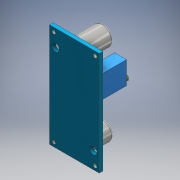
# Autodesk Inventor part: pcb_with_elements
Saved by Autodesk Inventor 2016 (Build 200138000, 138)
## iProperties
Created: 2016-10-13
Part Number: pcb_with_elements
Material: Generic
Document SubType Name: Modeling
Designer: Jakub
Density: 1 g/cm^3
Appearance: Default
Mass: 4.43836 g
Surface Area: 33.9944 cm^2
Volume: 4.43836 cm^3
Author: Jakub
Autodesk Inventor part; units mm, degrees
ref_plane "YZ Plane" through (0, 0, 0) normal (1, 0, 0) x (0, 1, 0)
ref_plane "XZ Plane" through (0, 0, 0) normal (0, 1, 0) x (-1, 0, 0)
ref_plane "XY Plane" through (0, 0, 0) normal (0, 0, 1) x (1, 0, 0)
sketch "Sketch1" plane through (0, 0, 0) normal (0, 1, 0) x (-1, 0, 0)
  line L0 (-10.375, 21.675) -> (10.375, 21.675)
  line L1 (10.375, 21.675) -> (10.375, -21.675)
  line L2 (10.375, -21.675) -> (-10.375, -21.675)
  line L3 (-10.375, -21.675) -> (-10.375, 21.675)
  line L4 (-10.375, 21.675) -> (10.375, -21.675) construction
  line L5 (10.375, 21.675) -> (-10.375, -21.675) construction
  point P0 (0, 0)
  dimension "d0" = 20.75
  dimension "d1" = 43.35
  constraints: 12 end point, 2 midpoint, 2 parallel, 1 horizontal, 1 perpendicular
  measures "d0" distance of L1.end L2.end
  measures "d1" distance of L0.end L1.end
extrude "Extrusion1" add sketch "Sketch1" along normal blind 1.5
sketch "Sketch2" plane through (0, 1.5, 0) normal (0, 1, 0) x (1, 0, 0)
  circle A0 centre (-8.625, -19.925) radius 0.75
  circle A1 centre (-8.625, 19.925) radius 0.75
  circle A2 centre (8.625, -19.925) radius 0.75
  circle A3 centre (8.625, 19.925) radius 0.75
  line L0 (-10.375, -21.675) -> (10.375, -21.675) projected
  line L1 (10.375, -21.675) -> (10.375, 21.675) projected
  line L2 (-10.375, 21.675) -> (-10.375, -21.675) projected
  line L3 (10.375, 21.675) -> (-10.375, 21.675) projected
  point P0 (0, 0)
  dimension "d4" = 1.5
  dimension "d5" = 1.5
  dimension "d6" = 1.5
  dimension "d7" = 1.5
  dimension "d8" = 1.75
  dimension "d9" = 1.75
  dimension "d10" = 1.75
  dimension "d11" = 1.75
  dimension "d12" = 1.75
  dimension "d13" = 1.75
  dimension "d14" = 1.75
  dimension "d15" = 1.75
  constraints: 4 centre point
  measures "d4" diameter of A0
  measures "d5" diameter of A1
  measures "d6" diameter of A2
  measures "d7" diameter of A3
  measures "d8" distance from line of L0 A2.centre
  measures "d9" distance from line of L1 A2.centre
  measures "d10" distance from line of L0 A0.centre
  measures "d11" distance from line of L2 A0.centre
  measures "d12" distance from line of L3 A1.centre
  measures "d13" distance from line of L2 A1.centre
  measures "d14" distance from line of L1 A3.centre
  measures "d15" distance from line of L3 A3.centre
extrude "Extrusion2" cut sketch "Sketch2" against normal up to next contours A0 | A1 | A2 | A3
sketch "Sketch3" plane through (0, 1.5, 0) normal (0, 1, 0) x (1, 0, 0)
  circle A0 centre (7.875, 14.675) radius 1.5
  circle A1 centre (-7.875, -14.675) radius 1.5
  line L0 (-10.375, 21.675) -> (-10.375, -21.675) projected
  line L1 (10.375, 21.675) -> (10.375, -21.675) projected
  line L2 (10.375, 21.675) -> (-10.375, 21.675) projected
  line L3 (-10.375, -21.675) -> (10.375, -21.675) projected
  point P0 (0, 0)
  dimension "d18" = 3
  dimension "d19" = 3
  dimension "d20" = 2.5
  dimension "d21" = 2.5
  dimension "d22" = 7
  dimension "d23" = 7
  constraints: 2 centre point
  measures "d18" diameter of A0
  measures "d19" diameter of A1
  measures "d20" distance from line of L0 A1.centre
  measures "d21" distance from line of L1 A0.centre
  measures "d22" distance from line of L2 A0.centre
  measures "d23" distance from line of L3 A1.centre
extrude "Extrusion3" cut sketch "Sketch3" against normal up to next contours A0 | A1
sketch "Sketch4" plane through (0, 1.5, 0) normal (0, 1, 0) x (1, 0, 0)
  line L0 (-7.125, -18.425) -> (-10.125, -18.425)
  line L1 (-10.125, -18.425) -> (-10.125, -21.425)
  line L2 (-10.125, -21.425) -> (-7.125, -21.425)
  line L3 (-7.125, -21.425) -> (-7.125, -18.425)
  circle A0 centre (-8.625, -19.925) radius 0.75 projected
  line L4 (-7.125, -18.425) -> (-10.125, -21.425) construction
  line L5 (-10.125, -18.425) -> (-7.125, -21.425) construction
  line L6 (10.125, -21.425) -> (7.125, -21.425)
  line L7 (7.125, -21.425) -> (7.125, -18.425)
  line L8 (7.125, -18.425) -> (10.125, -18.425)
  line L9 (10.125, -18.425) -> (10.125, -21.425)
  circle A1 centre (8.625, -19.925) radius 0.75 projected
  line L10 (10.125, -21.425) -> (7.125, -18.425) construction
  line L11 (7.125, -21.425) -> (10.125, -18.425) construction
  line L12 (7.125, 18.425) -> (10.125, 18.425)
  line L13 (10.125, 18.425) -> (10.125, 21.425)
  line L14 (10.125, 21.425) -> (7.125, 21.425)
  line L15 (7.125, 21.425) -> (7.125, 18.425)
  circle A2 centre (8.625, 19.925) radius 0.75 projected
  line L16 (7.125, 18.425) -> (10.125, 21.425) construction
  line L17 (10.125, 18.425) -> (7.125, 21.425) construction
  line L18 (-10.125, 21.425) -> (-7.125, 21.425)
  line L19 (-7.125, 21.425) -> (-7.125, 18.425)
  line L20 (-7.125, 18.425) -> (-10.125, 18.425)
  line L21 (-10.125, 18.425) -> (-10.125, 21.425)
  circle A3 centre (-8.625, 19.925) radius 0.75 projected
  line L22 (-10.125, 21.425) -> (-7.125, 18.425) construction
  line L23 (-7.125, 21.425) -> (-10.125, 18.425) construction
  circle A4 centre (-8.625, -19.925) radius 0.75
  circle A5 centre (8.625, -19.925) radius 0.75
  circle A6 centre (-8.625, 19.925) radius 0.75
  circle A7 centre (8.625, 19.925) radius 0.75
  point P0 (0, 0)
  dimension "d26" = 3
  dimension "d27" = 3
  dimension "d28" = 3
  dimension "d29" = 3
  dimension "d30" = 3
  dimension "d31" = 3
  dimension "d32" = 3
  dimension "d33" = 3
  constraints: 48 end point, 8 midpoint, 8 parallel, 4 centre point, 4 coincident, 4 concentric, 4 horizontal, 4 perpendicular
  measures "d26" distance of L2.end L1.end
  measures "d27" distance of L1.end L0.end
  measures "d28" distance of L7.end L8.end
  measures "d29" distance of L6.end L7.end
  measures "d30" distance of L14.end L13.end
  measures "d31" distance of L13.end L12.end
  measures "d32" distance of L19.end L20.end
  measures "d33" distance of L18.end L19.end
extrude "Extrusion4" add sketch "Sketch4" along normal blind 0.01
sketch "Sketch5" plane through (0, 1.5, 0) normal (0, 1, 0) x (1, 0, 0)
  circle A0 centre (0, 17.175) radius 4
  line L0 (10.375, 21.675) -> (-10.375, 21.675) projected
  point P0 (0, 0)
  dimension "d36" = 8
  dimension "d37" = 4.5
  constraints: 1 centre point
  measures "d36" diameter of A0
  measures "d37" distance from line of L0 A0.centre
extrude "Extrusion5" add sketch "Sketch5" along normal blind 11
sketch "Sketch6" plane through (0, 1.5, 0) normal (0, 1, 0) x (1, 0, 0)
  circle A0 centre (0, -17.175) radius 4
  line L0 (-10.375, -21.675) -> (10.375, -21.675) projected
  point P0 (0, 0)
  dimension "d40" = 8
  dimension "d41" = 4.5
  constraints: 1 centre point
  measures "d40" diameter of A0
  measures "d41" distance from line of L0 A0.centre
extrude "Extrusion6" add sketch "Sketch6" along normal blind 11
sketch "Sketch7" plane through (0, 1.5, 0) normal (0, 1, 0) x (1, 0, 0)
  line L0 (2.125, -12.175) -> (-9.875, -12.175)
  line L1 (-9.875, -12.175) -> (-9.875, -0.175)
  line L2 (-9.875, -0.175) -> (2.125, -0.175)
  line L3 (2.125, -0.175) -> (2.125, -12.175)
  line L4 (2.125, -12.175) -> (-9.875, -0.175) construction
  line L5 (-9.875, -12.175) -> (2.125, -0.175) construction
  line L6 (-10.375, 21.675) -> (-10.375, -21.675) projected
  circle A0 centre (0, -17.175) radius 4 projected
  point P0 (0, 0)
  point P1 (-3.875, -6.175)
  dimension "d44" = 12
  dimension "d45" = 12
  dimension "d46" = 0.5
  dimension "d47" = 5
  constraints: 12 end point, 2 midpoint, 2 parallel, 1 horizontal, 1 perpendicular
  measures "d44" distance of L1.end L2.end
  measures "d45" distance of L0.end L1.end
  measures "d46" distance between parallel lines of L6 L1
  measures "d47" distance from line of A0.centre L0
extrude "Extrusion7" add sketch "Sketch7" along normal blind 8 contours L0 L1 L2 L3
sketch "Sketch8" plane through (0, 9.5, 0) normal (0, 1, 0) x (1, 0, 0)
  line L0 (2.125, -12.175) -> (-9.875, -12.175) projected
  line L1 (-9.875, -12.175) -> (2.125, -0.175)
  circle A0 centre (-3.875, -6.175) radius 4.4338
  point P0 (0, 0)
  constraints: 2 end point, 1 centre point, 1 midpoint
extrude "Extrusion8" cut sketch "Sketch8" against normal blind 0.01
sketch "Sketch9" plane through (0, 1.5, 0) normal (0, 1, 0) x (1, 0, 0)
  line L0 (10.275, -13.675) -> (5.275, -13.675)
  line L1 (5.275, -13.675) -> (5.275, -4.175)
  line L2 (5.275, -4.175) -> (10.275, -4.175)
  line L3 (10.275, -4.175) -> (10.275, -13.675)
  line L4 (10.275, -13.675) -> (5.275, -4.175) construction
  line L5 (5.275, -13.675) -> (10.275, -4.175) construction
  line L6 (-10.375, -21.675) -> (10.375, -21.675) projected
  line L7 (10.375, 21.675) -> (10.375, -21.675) projected
  point P0 (0, 0)
  point P1 (7.775, -8.925)
  dimension "d52" = 5
  dimension "d53" = 9.5
  dimension "d54" = 8
  dimension "d55" = 0.1
  constraints: 12 end point, 2 midpoint, 2 parallel, 1 horizontal, 1 perpendicular
  measures "d52" distance of L1.end L2.end
  measures "d53" distance of L0.end L1.end
  measures "d54" distance between parallel lines of L6 L0
  measures "d55" distance between parallel lines of L7 L3
extrude "Extrusion9" add sketch "Sketch9" along normal blind 10
sketch "Sketch10" plane through (0, 11.5, 0) normal (0, 1, 0) x (1, 0, 0)
  circle A0 centre (8.775, -5.675) radius 1
  line L0 (10.275, -4.175) -> (5.275, -4.175) projected
  line L1 (10.275, -13.675) -> (10.275, -4.175) projected
  point P0 (0, 0)
  dimension "d58" = 2
  dimension "d59" = 1.5
  dimension "d60" = 1.5
  constraints: 1 centre point
  measures "d58" diameter of A0
  measures "d59" distance from line of L0 A0.centre
  measures "d60" distance from line of L1 A0.centre
extrude "Extrusion10" add sketch "Sketch10" along normal blind 1.5
sketch "Sketch11" plane through (8.775, 13, 5.675) normal (0, 1, 0) x (1, 0, 0)
  line L0 (1.224, -0.2665) -> (-1.224, -0.2665)
  line L1 (-1.224, -0.2665) -> (-1.224, 0.2665)
  line L2 (-1.224, 0.2665) -> (1.224, 0.2665)
  line L3 (1.224, 0.2665) -> (1.224, -0.2665)
  line L4 (1.224, -0.2665) -> (-1.224, 0.2665) construction
  line L5 (-1.224, -0.2665) -> (1.224, 0.2665) construction
  point P0 (-8.775, 5.675)
  point P1 (0, 0)
  constraints: 12 end point, 2 midpoint, 2 parallel, 1 horizontal, 1 perpendicular
extrude "Extrusion11" cut sketch "Sketch11" against normal blind 0.5
sketch "Sketch12" plane through (0, 1.5, 0) normal (0, 1, 0) x (1, 0, 0)
  line L0 (1.625, 1.325) -> (-6.875, 1.325)
  line L1 (-6.875, 1.325) -> (-6.875, 11.325)
  line L2 (-6.875, 11.325) -> (1.625, 11.325)
  line L3 (1.625, 11.325) -> (1.625, 1.325)
  line L4 (1.625, 1.325) -> (-6.875, 11.325) construction
  line L5 (-6.875, 1.325) -> (1.625, 11.325) construction
  line L6 (-10.375, 21.675) -> (-10.375, -21.675) projected
  line L7 (2.125, -0.175) -> (-9.875, -0.175) projected
  point P0 (0, 0)
  point P1 (-2.625, 6.325)
  dimension "d65" = 8.5
  dimension "d66" = 10
  dimension "d67" = 3.5
  dimension "d68" = 1.5
  constraints: 12 end point, 2 midpoint, 2 parallel, 1 horizontal, 1 perpendicular
  measures "d65" distance of L1.end L2.end
  measures "d66" distance of L0.end L1.end
  measures "d67" distance between parallel lines of L6 L1
  measures "d68" distance between parallel lines of L7 L0
extrude "Extrusion12" add sketch "Sketch12" along normal blind 4.5
sketch "Sketch13" plane through (1.625, 1.5, -1.325) normal (1, 0, 0) x (0, 0, -1)
  line L0 (10, 0) -> (0, 0) projected
  line L1 (0, 0) -> (1.5, 0)
  line L2 (1.5, 0) -> (1.5, 0.5)
  line L3 (1.5, 0.5) -> (0, 0.5)
  line L4 (0, 0.5) -> (0, 0)
  line L5 (10, 0) -> (8.5, 0)
  line L6 (8.5, 0) -> (8.5, 0.5)
  line L7 (8.5, 0.5) -> (10, 0.5)
  line L8 (10, 0.5) -> (10, 0)
  line L9 (2.12, 0) -> (3.62, 0)
  line L10 (3.62, 0) -> (3.62, 0.5)
  line L11 (3.62, 0.5) -> (2.12, 0.5)
  line L12 (2.12, 0.5) -> (2.12, 0)
  line L13 (6.38, 0) -> (7.88, 0)
  line L14 (7.88, 0) -> (7.88, 0.5)
  line L15 (7.88, 0.5) -> (6.38, 0.5)
  line L16 (6.38, 0.5) -> (6.38, 0)
  line L17 (4.24, 0) -> (5.74, 0)
  line L18 (5.74, 0) -> (5.74, 0.5)
  line L19 (5.74, 0.5) -> (4.24, 0.5)
  line L20 (4.24, 0.5) -> (4.24, 0)
  point P0 (-1.325, -1.5)
  dimension "d71" = 1.5
  dimension "d72" = 0.5
  dimension "d73" = 1.5
  dimension "d74" = 0.5
  dimension "d75" = 1.5
  dimension "d76" = 1.5
  dimension "d77" = 0.5
  dimension "d78" = 0.62
  dimension "d79" = 0.62
  dimension "d80" = 1.5
  dimension "d81" = 0.62
  constraints: 40 end point, 10 parallel, 5 horizontal, 5 perpendicular, 4 point on line
  measures "d71" distance of L3.end L2.end
  measures "d72" distance of L2.end L1.end
  measures "d73" distance of L6.end L7.end
  measures "d74" distance of L5.end L6.end
  measures "d75" distance of L11.end L10.end
  measures "d76" distance of L15.end L14.end
  measures "d77" distance of L14.end L13.end
  measures "d78" distance between parallel lines of L2 L12
  measures "d79" distance between parallel lines of L6 L14
  measures "d80" distance of L19.end L18.end
  measures "d81" distance between parallel lines of L10 L20
extrude "Extrusion13" add sketch "Sketch13" along normal blind 5
fillet "Fillet1" radius 1 6 edges at (2.125, 5.5, 12.175) (2.125, 5.5, 0.175) (-9.875, 5.5, 12.175) (-9.875, 5.5, 0.175) (-4, 12.5, 17.175) (-4, 12.5, -17.175)
body "Solid1"
